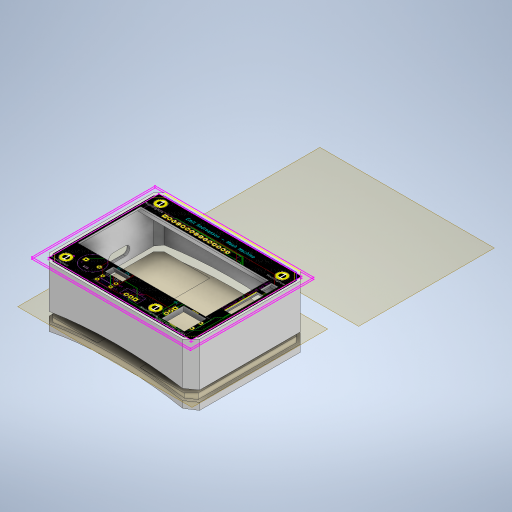
# Autodesk Inventor part: Mash Tank Box
Saved by Autodesk Inventor 2024 (Build 280153000, 153)
## iProperties
Created: 2024-11-04
Part Number: Mash Tank Box
Material: Generic
Document SubType Name: Modeling
Designer: Emil
Density: 1 g/cm^3
Appearance: Default
Author: Emil
Autodesk Inventor part; units mm, degrees
ref_plane "YZ Plane" through (0, 0, 0) normal (1, 0, 0) x (0, 1, 0)
ref_plane "XZ Plane" through (0, 0, 0) normal (0, 1, 0) x (-1, 0, 0)
sketch "Sketch21" plane through (0, 0, 0) normal (0, 1, 0) x (-1, 0, 0)
  line L0 (11.5687, 12.3265) -> (-78.4313, 12.3265)
  line L1 (-78.4313, 12.3265) -> (-78.4313, -57.6735)
  line L2 (-78.4313, -57.6735) -> (11.5687, -57.6735)
  line L3 (11.5687, -57.6735) -> (11.5687, 12.3265)
  line L4 (11.5687, 12.3265) -> (1.5687, 12.3265) construction
  line L5 (1.5687, -0.5983) -> (11.5687, -0.5983) construction
  line L6 (11.5687, -0.5985) -> (11.5687, 12.3265) projected
  point P0 (0, 0)
  dimension "d597" = 90
  dimension "d598" = 70
  constraints: 6 end point, 2 collinear, 2 horizontal, 1 parallel, 1 perpendicular, 3 other
  measures "d597" distance of L0.start L0.end
  measures "d598" distance of L0.end L1.end
extrude "Extrusion14" add sketch "Sketch21" along normal blind 1
ref_plane "Work Plane8" through (0, 40.25, 0) normal (0, 1, 0) x (1, 0, 0)
sketch "Sketch23" plane through (0, 40.25, 0) normal (0, 1, 0) x (1, 0, 0)
  line L0 (-11.5687, 57.6735) -> (-11.5687, -12.3265) projected
  line L1 (78.4313, -12.3265) -> (78.4313, 57.6735) projected
  line L2 (-11.5687, -12.3265) -> (78.4313, -12.3265) projected
  line L3 (-6.5487, 54.7786) -> (74.5546, 54.7786) construction
  line L4 (74.5546, 54.7786) -> (74.5546, -7.9714) construction
  line L5 (74.5546, -7.9714) -> (-6.5487, -7.9714) construction
  line L6 (-6.5487, -7.9714) -> (-6.5487, 54.7786) construction
  line L7 (-6.5487, 54.7786) -> (74.5546, 54.7786)
  line L8 (74.5546, 54.7786) -> (74.5546, -7.9714)
  line L9 (74.5546, -7.9714) -> (-6.5487, -7.9714)
  line L10 (-6.5487, -7.9714) -> (-6.5487, 54.7786)
  line L11 (-11.5687, 57.6735) -> (-11.5687, -12.3265) projected
  line L12 (-11.5687, -12.3265) -> (78.4313, -12.3265) projected
  line L13 (78.4313, -12.3265) -> (78.4313, 57.6735) projected
  line L14 (78.4313, 57.6735) -> (-11.5687, 57.6735) projected
  line L15 (-11.5687, 57.6735) -> (-11.5687, -12.3265) projected
  line L16 (-11.5687, -12.3265) -> (78.4313, -12.3265) projected
  line L17 (78.4313, -12.3265) -> (78.4313, 57.6735) projected
  line L18 (78.4313, 57.6735) -> (-11.5687, 57.6735) projected
  point P0 (0, 0)
  dimension "d668" = 62.75
  dimension "d724" = 81.1034
  constraints: 8 end point, 2 parallel, 1 horizontal, 1 perpendicular, 2 other
  measures "d668" distance of L3.end L4.end
  measures "d724" distance of L3.start L3.end
sketch3d "3D Sketch1"
decal "Decal3"
sketch "Sketch24" plane through (0, 1, 0) normal (0, 1, 0) x (1, 0, 0)
  line L0 (-3.7248, 55.2786) -> (71.0405, 55.2786)
  line L1 (71.0405, 55.2786) -> (75.0546, 51.2646)
  line L2 (71.0405, 55.2786) -> (76.7173, 55.2786) construction
  line L3 (75.0546, 51.2646) -> (75.0546, -4.4573)
  line L4 (75.0546, -4.4573) -> (71.0405, -8.4714)
  line L5 (71.0405, -8.4714) -> (-3.4649, -8.4714)
  line L6 (78.4313, -12.3265) -> (78.4313, 57.6735) projected
  line L7 (-3.4649, -8.4714) -> (-7.0487, -4.8875)
  line L8 (-7.0487, -4.8875) -> (-7.0487, 52.2952)
  line L9 (-7.0487, 52.2952) -> (-4.0653, 55.2786)
  line L10 (-4.0653, 55.2786) -> (-3.7248, 55.2786)
  line L11 (-11.5687, 57.6735) -> (-11.5687, -12.3265) projected
  line L12 (-11.5687, -12.3265) -> (78.4313, -12.3265) projected
  line L13 (78.4313, -12.3265) -> (78.4313, 57.6735) projected
  line L14 (78.4313, 57.6735) -> (-11.5687, 57.6735) projected
  line L15 (-11.5687, 57.6735) -> (-11.5687, -12.3265) projected
  line L16 (-11.5687, -12.3265) -> (78.4313, -12.3265) projected
  line L17 (78.4313, -12.3265) -> (78.4313, 57.6735) projected
  line L18 (78.4313, 57.6735) -> (-11.5687, 57.6735) projected
  line L19 (-11.5687, 57.6735) -> (-11.5687, -12.3265) projected
  line L20 (-11.5687, -12.3265) -> (78.4313, -12.3265) projected
  line L21 (78.4313, -12.3265) -> (78.4313, 57.6735) projected
  line L22 (78.4313, 57.6735) -> (-11.5687, 57.6735) projected
  line L23 (-6.5487, -7.9714) -> (-6.5487, 54.7786) projected
  line L24 (-6.5487, 54.7786) -> (74.5546, 54.7786) projected
  line L25 (74.5546, 54.7786) -> (74.5546, -7.9714) construction
  line L26 (74.5546, -7.9714) -> (-6.5487, -7.9714) projected
  line L27 (-4.0653, 56.7786) -> (71.718, 56.7786)
  line L28 (71.718, 56.7786) -> (76.5546, 51.942)
  line L29 (76.5546, 51.942) -> (76.5546, -5.1544)
  line L30 (76.5546, -5.1544) -> (71.7377, -9.9714)
  line L31 (71.7377, -9.9714) -> (-4.1146, -9.9714)
  line L32 (-4.1146, -9.9714) -> (-8.5487, -5.5372)
  line L33 (-8.5487, -5.5372) -> (-8.5487, 53.5846)
  line L34 (-8.5487, 53.5846) -> (-5.3547, 56.7786)
  line L35 (-5.3547, 56.7786) -> (-4.0653, 56.7786)
  point P0 (0, 0)
  point P1 (71.5405, 54.7786)
  point P2 (73.718, 54.7786)
  point P3 (-6.5487, -7.5372)
  point P4 (-6.5487, -5.3875)
  point P5 (-6.5487, 52.7952)
  point P6 (-4.5653, 54.7786)
  dimension "d681" = 45
  dimension "d682" = 135
  dimension "d683" = 135
  dimension "d684" = 135
  dimension "d685" = 0.5
  dimension "d686" = 0.5
  dimension "d687" = 0.5
  dimension "d688" = 0.5
  dimension "d693" = 135
  dimension "d694" = 135
  dimension "d695" = 135
  dimension "d696" = 135
  dimension "d697" = 1.5
  dimension "d698" = 1.5
  dimension "d699" = 1.5
  dimension "d700" = 1.5
  constraints: 38 end point, 3 parallel, 3 perpendicular, 2 collinear, 2 horizontal, 1 equal length, 1 point on line, 1 vertical
  measures "d681" angle of L1 L2
  measures "d682" angle of L3 L4
  measures "d683" angle of L5 L7
  measures "d684" angle of L8 L9
  measures "d685" distance between parallel lines of L8 L23
  measures "d686" distance between parallel lines of L0 L24
  measures "d687" distance between parallel lines of L3 L25
  measures "d688" distance between parallel lines of L26 L5
  measures "d693" angle of L27 L28
  measures "d694" angle of L29 L30
  measures "d695" angle of L31 L32
  measures "d696" angle of L33 L34
  measures "d697" distance between parallel lines of L27 L0
  measures "d698" distance between parallel lines of L33 L8
  measures "d699" distance between parallel lines of L29 L3
  measures "d700" distance between parallel lines of L5 L31
extrude "Extrusion16" add sketch "Sketch24" against normal blind 25 contours L10 L9 L24 L23 L8 L7 L32 L33 L34 L35 L27 L28 L1 L0 | L24 L28 L29 L30 L26 L4 L3 L1 | L9 L23 L24 | L7 L26 L32 L23 | L26 L30 L31 L32 L7 L5 L4
sketch "Sketch25" plane through (0, 1, 0) normal (0, 1, 0) x (1, 0, 0)
  line L0 (-5.323, 43.3544) -> (67.1649, 43.3544)
  line L1 (67.1649, 43.3544) -> (67.1649, 7.6379)
  line L2 (67.1649, 7.6379) -> (-5.323, 7.6379)
  line L3 (-5.323, 7.6379) -> (-5.323, 43.3544)
  line L4 (55.553, 6.7561) -> (68.4085, 6.7561)
  line L5 (68.4085, 6.7561) -> (68.4085, -5.6618)
  line L6 (68.4085, -5.6618) -> (55.553, -5.6618)
  line L7 (55.553, -5.6618) -> (55.553, 6.7561)
  line L8 (16.4334, 5.9938) -> (26.351, 5.9938)
  line L9 (26.351, 5.9938) -> (26.351, 1.2764)
  line L10 (26.351, 1.2764) -> (16.4334, 1.2764)
  line L11 (16.4334, 1.2764) -> (16.4334, 5.9938)
  line L12 (69.3512, 42.8492) -> (73.1491, 42.8492)
  line L13 (73.1491, 42.8492) -> (73.1491, 36.4177)
  line L14 (73.1491, 36.4177) -> (69.3512, 36.4177)
  line L15 (69.3512, 36.4177) -> (69.3512, 42.8492)
  line L16 (69.3512, 34.3565) -> (73.3289, 34.3565)
  line L17 (73.3289, 34.3565) -> (73.3289, 16.0733)
  line L18 (73.3289, 16.0733) -> (69.3512, 16.0733)
  line L19 (69.3512, 16.0733) -> (69.3512, 34.3565)
  point P0 (0, 0)
  point P1 (73.1491, 16.0733)
  constraints: 40 end point, 10 parallel, 5 horizontal, 5 perpendicular, 2 point on line
extrude "Extrusion17" cut sketch "Sketch25" against normal up to surface (1 mm away)
sketch "Sketch26" plane through (0, 1, 0) normal (0, 1, 0) x (1, 0, 0)
  circle A0 centre (-1.179, 50.5743) radius 1.25
  circle A1 centre (68.8579, 49.4155) radius 1.25
  circle A2 centre (48.6287, -2.2236) radius 1.25
  circle A3 centre (-1.6747, -2.72) radius 1.25
  point P0 (0, 0)
  dimension "d707" = 2.5
  dimension "d708" = 2.5
  dimension "d709" = 2.5
  dimension "d710" = 2.5
  constraints: 4 centre point
  measures "d707" diameter of A0
  measures "d708" diameter of A1
  measures "d709" diameter of A2
  measures "d710" diameter of A3
extrude "Extrusion18" add sketch "Sketch26" against normal blind 8
sketch "Sketch27" plane through (0, 0, 0) normal (0, -1, 0) x (1, 0, 0)
  line L0 (-8.5487, -53.5846) -> (-5.3547, -56.7786) projected
  line L1 (-8.5487, -53.5846) -> (-5.3547, -56.7786)
  line L2 (71.718, -56.7786) -> (76.5546, -51.942) projected
  line L3 (-5.3547, -56.7786) -> (71.718, -56.7786)
  line L4 (71.718, -56.7786) -> (76.5546, -51.942)
  line L5 (76.5546, -51.942) -> (76.5546, 4.0683)
  line L6 (76.5546, 5.1544) -> (71.7377, 9.9714) projected
  line L7 (71.7377, 9.9714) -> (-4.1146, 9.9714)
  line L8 (-8.5487, 5.5372) -> (-8.5487, -53.5846) projected
  line L9 (-4.1146, 9.9714) -> (-8.5487, 5.5372)
  line L10 (-8.5487, 5.5372) -> (-8.5487, -53.5846)
  line L11 (-8.5487, -53.5846) -> (-5.3547, -56.7786)
  line L12 (78.4313, -57.6735) -> (-11.5687, -57.6735) projected
  line L13 (-11.5687, -57.6735) -> (78.4313, -57.6735)
  line L14 (78.4313, -57.6735) -> (78.4313, 12.3265)
  line L15 (78.4313, 12.3265) -> (-11.5687, 12.3265)
  line L16 (-11.5687, 12.3265) -> (-11.5687, -57.6735)
  line L17 (76.5546, -51.942) -> (76.5546, 5.1544) projected
  line L18 (76.5546, 4.0683) -> (76.5546, 5.1544)
  line L19 (76.5546, 5.1544) -> (71.7377, 9.9714)
  point P0 (0, 0)
  constraints: 28 end point, 6 collinear, 3 parallel, 3 perpendicular, 2 horizontal
sketch "Sketch28" plane through (-8.5487, 1, -53.5846) normal (-1, 0, 0) x (0, 0, 1)
  line L0 (14.806, -19.1) -> (26.806, -19.1) construction
  line L1 (17.306, -21.6) -> (24.306, -21.6)
  line L2 (24.306, -16.6) -> (17.306, -16.6)
  arc A0 (17.306, -16.6) -> (17.306, -21.6) centre (17.306, -19.1) ccw
  arc A1 (24.306, -21.6) -> (24.306, -16.6) centre (24.306, -19.1) ccw
  line L3 (0, 0) -> (59.1218, 0) projected
  line L4 (-3.194, -25) -> (-3.194, 0) projected
  line L5 (61.556, 0) -> (-1.194, 0) projected
  line L6 (-1.694, -1) -> (-1.694, -25) projected
  line L7 (58.4722, -1) -> (1.2894, -1) projected
  point P0 (53.5846, -1)
  point P1 (20.806, -19.1)
  point P2 (-1.694, -13)
  dimension "d715" = 12
  dimension "d716" = 5
  dimension "d721" = 18.1
  dimension "d733" = 24
  constraints: 8 end point, 7 point on circle, 4 tangent, 2 centre point, 2 midpoint, 2 point on line, 1 horizontal, 1 parallel
  measures "d715" distance of L0.start L0.end
  measures "d716" diameter of A1
  measures "d721" distance from line of L7 point (20.806, -19.1)
  measures "d733" distance from line of L4 point (20.806, -19.1)
extrude "Extrusion20" cut sketch "Sketch28" against normal blind 10
extrude "Extrusion21" cut sketch "Sketch27" against normal blind 25
sketch "Sketch29" plane through (0, 0, 0) normal (0, -1, 0) x (1, 0, 0)
  line L0 (-5.3371, -7.6383) -> (-7.0487, -7.6383) construction
  line L1 (-7.0487, 4.8875) -> (-7.0487, -52.2952) construction
  line L2 (68.4085, -6.7561) -> (68.4085, 5.6618) projected
  line L3 (-7.0487, -7.6383) -> (68.4085, -7.6383)
  line L4 (68.4085, -7.6383) -> (68.4085, -6.7561)
  line L5 (68.4085, -6.7561) -> (-7.0487, -6.7561)
  line L6 (-7.0487, -6.7561) -> (-7.0487, -7.6383)
  line L7 (75.0546, 4.4573) -> (75.0546, -51.2646) projected
  line L8 (68.4085, -7.6383) -> (75.0546, -7.6383)
  line L9 (75.0546, -7.6383) -> (75.0546, -6.7561)
  line L10 (75.0546, -6.7561) -> (68.4085, -6.7561)
  line L11 (68.4085, -6.7561) -> (68.4085, -7.6383)
  line L12 (-5.3371, -43.3314) -> (-7.0487, -43.3314) construction
  line L13 (-7.0487, -43.3314) -> (75.0546, -43.3314)
  line L14 (75.0546, -43.3314) -> (75.0546, -44.3314)
  line L15 (75.0546, -44.3314) -> (-7.0487, -44.3314)
  line L16 (-7.0487, -44.3314) -> (-7.0487, -43.3314)
  line L17 (67.165, -7.6383) -> (68.165, -7.6383)
  line L18 (68.165, -7.6383) -> (68.165, -43.3314)
  line L19 (68.165, -43.3314) -> (67.165, -43.3314)
  line L20 (67.165, -43.3314) -> (67.165, -7.6383)
  line L21 (55.553, -6.7561) -> (55.553, 5.6618) projected
  line L22 (-3.4649, 8.4714) -> (71.0405, 8.4714) projected
  line L23 (55.553, -6.7561) -> (54.553, -6.7561)
  line L24 (54.553, -6.7561) -> (54.553, 8.4714)
  line L25 (54.553, 8.4714) -> (55.553, 8.4714)
  line L26 (55.553, 8.4714) -> (55.553, -6.7561)
  line L27 (16.4334, -6.7561) -> (15.4334, -6.7561)
  line L28 (15.4334, -6.7561) -> (15.4334, 8.4714)
  line L29 (15.4334, 8.4714) -> (16.4334, 8.4714)
  line L30 (16.4334, 8.4714) -> (16.4334, -6.7561)
  line L31 (-4.0653, -55.2786) -> (71.0405, -55.2786) projected
  line L32 (31.6564, -44.3314) -> (32.6564, -44.3314)
  line L33 (32.6564, -44.3314) -> (32.6564, -55.2786)
  line L34 (32.6564, -55.2786) -> (31.6564, -55.2786)
  line L35 (31.6564, -55.2786) -> (31.6564, -44.3314)
  point P0 (0, 0)
  point P1 (55.553, 5.6618)
  dimension "d730" = 1
  dimension "d731" = 1
  dimension "d738" = 1
  dimension "d739" = 1
  dimension "d740" = 1
  constraints: 60 end point, 14 parallel, 12 point on line, 8 horizontal, 8 perpendicular
  measures "d730" distance of L13.end L14.end
  measures "d731" distance of L18.end L19.end
  measures "d738" distance of L24.end L25.end
  measures "d739" distance of L28.end L29.end
  measures "d740" distance of L33.end L34.end
extrude "Extrusion22" add sketch "Sketch29" along normal blind 2 contours L6 L5 L4 L3 | L3 L18 L13 L20 | L13 L7 L15 L16 | L28 L22 L30 L5 | L4 L10 L7 L8 | L24 L22 L26 L21 L5 | L15 L33 L31 L35
sketch "Sketch30" plane through (-4.1146, 1, 9.9714) normal (0, 0, 1) x (1, 0, 0)
  line L0 (-4.4341, -25) -> (-4.4341, 0) projected
  line L1 (80.6692, -25) -> (80.6692, 0) projected
  line L2 (-4.4341, -25) -> (-1.2401, -25) projected
  arc A0 (80.6692, -25) -> (-4.4341, -25) centre (38.1176, -261.1977) ccw
  line L3 (-4.4341, -25) -> (80.6692, -25)
  line L4 (79.1692, -1) -> (79.1692, -25) projected
  point P0 (4.1146, -1)
  dimension "d735" = 240
  constraints: 2 end point, 2 point on circle, 1 centre point, 1 perpendicular
  measures "d735" radius of A0
extrude "Extrusion23" cut sketch "Sketch30" against normal through all
sketch "Sketch31" plane through (0, 1, 0) normal (0, 1, 0) x (1, 0, 0)
  line L0 (-3.4649, -8.4714) -> (71.0405, -8.4714) projected
  line L1 (75.0546, -4.4573) -> (71.0405, -8.4714) projected
  line L2 (-3.4649, -8.4714) -> (71.0405, -8.4714)
  line L3 (71.0405, -8.4714) -> (75.0546, -4.4573)
  line L4 (75.0546, -4.4573) -> (75.0546, 51.258)
  line L5 (69.3512, 16.0733) -> (69.3512, 34.3565) projected
  line L6 (75.0546, 51.258) -> (71.0405, 55.2721)
  line L7 (71.0405, 55.2721) -> (-4.0719, 55.2721)
  line L8 (71.718, 56.7786) -> (-5.3547, 56.7786) projected
  line L9 (-7.0487, 44.3314) -> (-7.0487, 52.2952) projected
  line L10 (-4.0719, 55.2721) -> (-7.0487, 52.2952)
  line L11 (-7.0487, 52.2952) -> (-7.0487, -4.8875)
  line L12 (-7.0487, -4.8875) -> (-3.4649, -8.4714) projected
  line L13 (-3.4649, -8.4714) -> (-7.0487, -4.8875)
  constraints: 16 end point, 3 collinear, 3 parallel, 1 horizontal
ref_plane "Work Plane10" through (-8.5487, -24, -53.5846) normal (0, 1, 0) x (0, 0, -1)
sketch "Sketch32" plane through (-8.5487, -24, -53.5846) normal (0, 1, 0) x (0, 0, -1)
  line L0 (3.194, -80.2667) -> (3.194, -3.194) projected
  line L1 (-58.7391, -85.1034) -> (-1.6426, -85.1034) projected
  line L2 (-63.556, -4.4341) -> (-63.556, -80.2865) projected
  line L3 (-63.556, -4.4341) -> (-63.556, -80.2865)
  line L4 (-58.7391, -85.1034) -> (-63.556, -80.2865) projected
  line L5 (-63.556, -80.2865) -> (-58.7391, -85.1034)
  line L6 (-58.7391, -85.1034) -> (-1.6426, -85.1034)
  line L7 (-1.6426, -85.1034) -> (3.194, -80.2667) projected
  line L8 (3.194, -80.2667) -> (-1.6426, -85.1034)
  line L9 (-1.6426, -85.1034) -> (3.194, -80.2667)
  line L10 (3.194, -80.2667) -> (3.194, -3.194)
  line L11 (3.194, -3.194) -> (0, 0) projected
  line L12 (3.194, -3.194) -> (0, 0)
  line L13 (-59.1218, 0) -> (-63.556, -4.4341) projected
  line L14 (0, 0) -> (-59.1218, 0)
  line L15 (-59.1218, 0) -> (-63.556, -4.4341)
  line L16 (-63.556, -80.2865) -> (-63.556, -4.4341) projected
  line L17 (-63.556, -4.4341) -> (-63.556, -80.2865)
  point P0 (-53.5846, -8.5487)
  constraints: 20 end point, 8 collinear, 2 horizontal
extrude "Extrusion24" add sketch "Sketch32" against normal blind 10 separate body
sketch "Sketch33" plane through (-4.1146, -24, 9.9714) normal (0, 0, 1) x (1, 0, 0)
  line L0 (80.6692, 0) -> (80.6692, -10) projected
  line L1 (0, -10) -> (-4.4341, -10) projected
  arc A0 (80.6692, -10) -> (-4.4341, -10) centre (38.1176, -205.421) ccw
  line L2 (-4.4341, 0) -> (-4.4341, -10) projected
  line L3 (-4.4341, -10) -> (-4.4341, -6)
  arc A1 (80.6692, -6) -> (-4.4341, -6) centre (38.1176, -242.1977) ccw
  line L4 (-25.4541, 0) -> (100.5459, 0) projected
  line L5 (75.8523, -10) -> (0, -10) projected
  line L6 (-4.4341, -6) -> (-4.4341, 0)
  line L7 (-4.4341, 0) -> (80.6692, 0)
  line L8 (80.6692, -5.7262) -> (80.6692, 0)
  line L9 (80.6692, -10) -> (-4.4341, -10)
  point P0 (4.1146, 24)
  dimension "d746" = 4
  dimension "d747" = 240
  constraints: 10 end point, 4 point on circle, 3 collinear, 3 point on line, 2 centre point, 1 perpendicular
  measures "d746" distance of L1.end L3.end
  measures "d747" radius of A1
extrude "Extrusion25" cut sketch "Sketch33" against normal up to surface (66.75 mm away) contours L0 A1 L2 L4 | L9 L5 L1 A0 bodies 2
ref_plane "Work Plane11" through (76.5546, -30, 9.9714) normal (0, 1, 0) x (0, 0, 1)
sketch "Sketch34" plane through (76.5546, -30, 9.9714) normal (0, 1, 0) x (0, 0, 1)
  line L0 (-65.2434, -80.6265) -> (-62.2665, -83.6034) projected
  line L1 (-54.3027, -83.6034) -> (-62.2665, -83.6034) projected
  line L2 (-65.2434, -5.5141) -> (-65.2434, -80.6265) projected
  line L3 (-61.2294, -1.5) -> (-65.2434, -5.5141) projected
  line L4 (-5.5141, -1.5) -> (-61.2294, -1.5) projected
  line L5 (-5.5141, -1.5) -> (-1.5, -5.5141) projected
  line L6 (-1.5, -80.0196) -> (-1.5, -5.5141) projected
  line L7 (-5.0838, -83.6034) -> (-1.5, -80.0196) projected
  line L8 (-62.2665, -83.6034) -> (-65.2434, -80.6265)
  line L9 (-65.2434, -80.6265) -> (-65.2434, -5.5141)
  line L10 (-65.2434, -5.5141) -> (-61.2294, -1.5)
  line L11 (-61.2294, -1.5) -> (-5.5141, -1.5)
  line L12 (-5.5141, -1.5) -> (-1.5, -5.5141)
  line L13 (-1.5, -5.5141) -> (-1.5, -80.0196)
  line L14 (-1.5, -80.0196) -> (-5.0838, -83.6034)
  line L15 (-5.0838, -83.6034) -> (-62.2665, -83.6034)
  line L16 (-62.2665, -83.6034) -> (-65.2434, -80.6265)
  point P0 (-9.9714, -76.5546)
  constraints: 18 end point, 7 collinear, 1 vertical
extrude "Extrusion26" add sketch "Sketch34" along normal blind 3.5 bodies 2
sketch "Sketch35" plane through (-4.1146, -33.0869, 9.9714) normal (0, 0, 1) x (1, 0, 0)
  arc A0 (80.6692, -0.9131) -> (75.8523, 0.0739) centre (38.1176, -196.334) ccw projected
  arc A1 (-1.2401, -0.2448) -> (-4.4341, -0.9131) centre (38.1176, -196.334) ccw projected
  arc A2 (80.6692, -0.9131) -> (-4.4341, -0.9131) centre (38.1176, -196.334) ccw
  line L0 (-4.4341, -0.9131) -> (80.6692, -0.9131)
  line L1 (-4.4341, 3.0869) -> (-4.4341, -0.9131) projected
  point P0 (4.1146, 33.0869)
  point P1 (75.8523, 0.0739)
  constraints: 2 end point, 2 point on circle, 1 centre point, 1 perpendicular
extrude "Extrusion27" cut sketch "Sketch35" against normal up to surface (66.75 mm away) bodies 2
body "Solid8"
body "Solid9"
